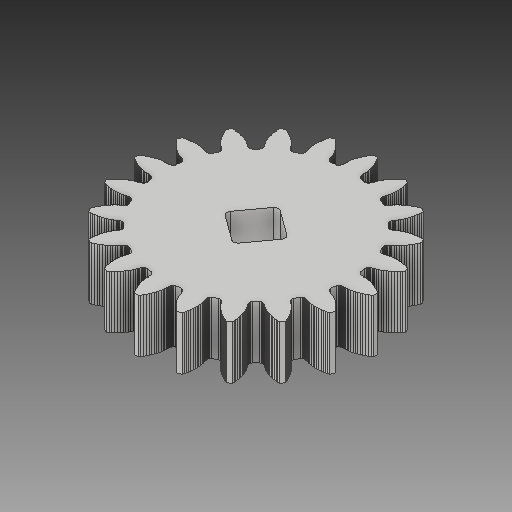
# Autodesk Inventor part: gear20
Saved by Autodesk Inventor 2019 (Build 230136000, 136)
## iProperties
Created: 2018-12-28
Part Number: gear20
Material: Generic
Document SubType Name: Modeling
Designer: Varga Daniel
Density: 1 g/cm^3
Appearance: Default
Sending System: SolidWorks 2018
Last Author: david
Last Saved: 2018-12-28
Author: Varga Daniel
Autodesk Inventor part; units mm, degrees
ref_plane "YZ Plane" through (0, 0, 0) normal (1, 0, 0) x (0, 1, 0)
ref_plane "XZ Plane" through (0, 0, 0) normal (0, 1, 0) x (-1, 0, 0)
ref_plane "XY Plane" through (0, 0, 0) normal (0, 0, 1) x (1, 0, 0)
sketch "Sketch1" plane through (0, 0, 0) normal (0, 1, 0) x (-1, 0, 0)
  line L0 (19.9269, 12.3554) -> (19.9815, 12.2461)
  line L1 (19.9815, 12.2461) -> (20.0271, 12.2067)
  line L2 (20.0271, 12.2067) -> (20.0711, 12.1796)
  line L3 (20.0711, 12.1796) -> (20.1144, 12.1591)
  line L4 (20.1144, 12.1591) -> (20.1571, 12.1432)
  line L5 (20.1571, 12.1432) -> (20.2414, 12.1206)
  line L6 (20.2414, 12.1206) -> (20.3248, 12.107)
  line L7 (20.3248, 12.107) -> (20.4075, 12.1)
  line L8 (20.4075, 12.1) -> (20.4897, 12.0984)
  line L9 (20.4897, 12.0984) -> (20.6534, 12.1025)
  line L10 (20.6534, 12.1025) -> (20.8187, 12.0882)
  line L11 (20.8187, 12.0882) -> (20.9851, 12.06)
  line L12 (20.9851, 12.06) -> (21.1522, 12.0208)
  line L13 (21.1522, 12.0208) -> (21.3198, 11.9721)
  line L14 (21.3198, 11.9721) -> (21.4876, 11.9147)
  line L15 (21.4876, 11.9147) -> (21.6554, 11.8491)
  line L16 (21.6554, 11.8491) -> (21.823, 11.7758)
  line L17 (21.823, 11.7758) -> (21.9904, 11.695)
  line L18 (21.9904, 11.695) -> (22.1573, 11.6069)
  line L19 (22.1573, 11.6069) -> (22.3236, 11.5119)
  line L20 (22.3236, 11.5119) -> (22.4478, 11.4361)
  line L21 (22.4478, 11.4361) -> (22.4478, 11.0137)
  line L22 (22.4478, 11.0137) -> (22.3236, 10.9379)
  line L23 (22.3236, 10.9379) -> (22.1573, 10.8429)
  line L24 (22.1573, 10.8429) -> (21.9904, 10.7549)
  line L25 (21.9904, 10.7549) -> (21.823, 10.6741)
  line L26 (21.823, 10.6741) -> (21.6554, 10.6007)
  line L27 (21.6554, 10.6007) -> (21.4876, 10.5351)
  line L28 (21.4876, 10.5351) -> (21.3198, 10.4777)
  line L29 (21.3198, 10.4777) -> (21.1522, 10.429)
  line L30 (21.1522, 10.429) -> (20.9851, 10.3898)
  line L31 (20.9851, 10.3898) -> (20.8187, 10.3616)
  line L32 (20.8187, 10.3616) -> (20.6534, 10.3473)
  line L33 (20.6534, 10.3473) -> (20.4897, 10.3514)
  line L34 (20.4897, 10.3514) -> (20.4075, 10.3498)
  line L35 (20.4075, 10.3498) -> (20.3248, 10.3428)
  line L36 (20.3248, 10.3428) -> (20.2414, 10.3292)
  line L37 (20.2414, 10.3292) -> (20.1571, 10.3066)
  line L38 (20.1571, 10.3066) -> (20.1144, 10.2907)
  line L39 (20.1144, 10.2907) -> (20.0711, 10.2703)
  line L40 (20.0711, 10.2703) -> (20.0271, 10.2431)
  line L41 (20.0271, 10.2431) -> (19.9815, 10.2037)
  line L42 (19.9815, 10.2037) -> (19.9269, 10.0944)
  line L43 (19.9269, 10.0944) -> (19.8503, 9.611)
  line L44 (19.8503, 9.611) -> (19.8685, 9.4902)
  line L45 (19.8685, 9.4902) -> (19.8997, 9.4386)
  line L46 (19.8997, 9.4386) -> (19.9332, 9.3992)
  line L47 (19.9332, 9.3992) -> (19.968, 9.3664)
  line L48 (19.968, 9.3664) -> (20.0037, 9.338)
  line L49 (20.0037, 9.338) -> (20.0769, 9.2905)
  line L50 (20.0769, 9.2905) -> (20.152, 9.2518)
  line L51 (20.152, 9.2518) -> (20.2285, 9.2196)
  line L52 (20.2285, 9.2196) -> (20.3062, 9.1927)
  line L53 (20.3062, 9.1927) -> (20.4631, 9.146)
  line L54 (20.4631, 9.146) -> (20.6159, 9.0813)
  line L55 (20.6159, 9.0813) -> (20.7655, 9.003)
  line L56 (20.7655, 9.003) -> (20.9123, 8.9141)
  line L57 (20.9123, 8.9141) -> (21.0566, 8.8161)
  line L58 (21.0566, 8.8161) -> (21.1984, 8.7096)
  line L59 (21.1984, 8.7096) -> (21.3378, 8.5954)
  line L60 (21.3378, 8.5954) -> (21.4746, 8.4738)
  line L61 (21.4746, 8.4738) -> (21.6088, 8.3452)
  line L62 (21.6088, 8.3452) -> (21.7403, 8.2099)
  line L63 (21.7403, 8.2099) -> (21.8691, 8.0681)
  line L64 (21.8691, 8.0681) -> (21.9638, 7.9577)
  line L65 (21.9638, 7.9577) -> (21.8333, 7.556)
  line L66 (21.8333, 7.556) -> (21.6917, 7.5223)
  line L67 (21.6917, 7.5223) -> (21.5042, 7.4833)
  line L68 (21.5042, 7.4833) -> (21.3183, 7.4511)
  line L69 (21.3183, 7.4511) -> (21.1341, 7.426)
  line L70 (21.1341, 7.426) -> (20.952, 7.4081)
  line L71 (20.952, 7.4081) -> (20.7721, 7.3976)
  line L72 (20.7721, 7.3976) -> (20.5948, 7.3948)
  line L73 (20.5948, 7.3948) -> (20.4204, 7.4002)
  line L74 (20.4204, 7.4002) -> (20.2493, 7.4146)
  line L75 (20.2493, 7.4146) -> (20.0824, 7.4392)
  line L76 (20.0824, 7.4392) -> (19.9207, 7.4767)
  line L77 (19.9207, 7.4767) -> (19.7663, 7.5312)
  line L78 (19.7663, 7.5312) -> (19.6877, 7.555)
  line L79 (19.6877, 7.555) -> (19.6068, 7.5739)
  line L80 (19.6068, 7.5739) -> (19.5233, 7.5868)
  line L81 (19.5233, 7.5868) -> (19.4362, 7.5914)
  line L82 (19.4362, 7.5914) -> (19.3906, 7.5894)
  line L83 (19.3906, 7.5894) -> (19.3432, 7.5834)
  line L84 (19.3432, 7.5834) -> (19.2929, 7.5712)
  line L85 (19.2929, 7.5712) -> (19.2373, 7.5477)
  line L86 (19.2373, 7.5477) -> (19.1516, 7.4607)
  line L87 (19.1516, 7.4607) -> (18.9294, 7.0246)
  line L88 (18.9294, 7.0246) -> (18.9094, 6.9041)
  line L89 (18.9094, 6.9041) -> (18.9231, 6.8454)
  line L90 (18.9231, 6.8454) -> (18.9428, 6.7976)
  line L91 (18.9428, 6.7976) -> (18.9657, 6.7556)
  line L92 (18.9657, 6.7556) -> (18.9909, 6.7176)
  line L93 (18.9909, 6.7176) -> (19.0459, 6.6498)
  line L94 (19.0459, 6.6498) -> (19.1054, 6.5898)
  line L95 (19.1054, 6.5898) -> (19.1682, 6.5355)
  line L96 (19.1682, 6.5355) -> (19.2337, 6.4859)
  line L97 (19.2337, 6.4859) -> (19.3685, 6.393)
  line L98 (19.3685, 6.393) -> (19.4938, 6.2843)
  line L99 (19.4938, 6.2843) -> (19.6119, 6.1636)
  line L100 (19.6119, 6.1636) -> (19.7241, 6.0337)
  line L101 (19.7241, 6.0337) -> (19.831, 5.8958)
  line L102 (19.831, 5.8958) -> (19.933, 5.7507)
  line L103 (19.933, 5.7507) -> (20.0302, 5.599)
  line L104 (20.0302, 5.599) -> (20.1228, 5.4411)
  line L105 (20.1228, 5.4411) -> (20.2107, 5.2774)
  line L106 (20.2107, 5.2774) -> (20.294, 5.1081)
  line L107 (20.294, 5.1081) -> (20.3726, 4.9334)
  line L108 (20.3726, 4.9334) -> (20.4286, 4.7991)
  line L109 (20.4286, 4.7991) -> (20.1803, 4.4574)
  line L110 (20.1803, 4.4574) -> (20.0353, 4.4691)
  line L111 (20.0353, 4.4691) -> (19.8449, 4.4899)
  line L112 (19.8449, 4.4899) -> (19.6581, 4.5168)
  line L113 (19.6581, 4.5168) -> (19.4752, 4.5498)
  line L114 (19.4752, 4.5498) -> (19.2964, 4.589)
  line L115 (19.2964, 4.589) -> (19.1221, 4.6346)
  line L116 (19.1221, 4.6346) -> (18.9526, 4.6868)
  line L117 (18.9526, 4.6868) -> (18.7885, 4.7459)
  line L118 (18.7885, 4.7459) -> (18.6302, 4.8124)
  line L119 (18.6302, 4.8124) -> (18.479, 4.8874)
  line L120 (18.479, 4.8874) -> (18.3369, 4.973)
  line L121 (18.3369, 4.973) -> (18.2069, 5.0725)
  line L122 (18.2069, 5.0725) -> (18.1394, 5.1195)
  line L123 (18.1394, 5.1195) -> (18.0684, 5.1625)
  line L124 (18.0684, 5.1625) -> (17.9929, 5.2005)
  line L125 (17.9929, 5.2005) -> (17.9114, 5.2318)
  line L126 (17.9114, 5.2318) -> (17.8675, 5.244)
  line L127 (17.8675, 5.244) -> (17.8205, 5.2529)
  line L128 (17.8205, 5.2529) -> (17.7689, 5.2568)
  line L129 (17.7689, 5.2568) -> (17.7089, 5.2517)
  line L130 (17.7089, 5.2517) -> (17.6005, 5.1954)
  line L131 (17.6005, 5.1954) -> (17.2544, 4.8494)
  line L132 (17.2544, 4.8494) -> (17.1981, 4.7409)
  line L133 (17.1981, 4.7409) -> (17.193, 4.6809)
  line L134 (17.193, 4.6809) -> (17.1969, 4.6293)
  line L135 (17.1969, 4.6293) -> (17.2058, 4.5823)
  line L136 (17.2058, 4.5823) -> (17.218, 4.5384)
  line L137 (17.218, 4.5384) -> (17.2493, 4.4569)
  line L138 (17.2493, 4.4569) -> (17.2873, 4.3814)
  line L139 (17.2873, 4.3814) -> (17.3303, 4.3104)
  line L140 (17.3303, 4.3104) -> (17.3773, 4.2429)
  line L141 (17.3773, 4.2429) -> (17.4768, 4.113)
  line L142 (17.4768, 4.113) -> (17.5624, 3.9708)
  line L143 (17.5624, 3.9708) -> (17.6374, 3.8196)
  line L144 (17.6374, 3.8196) -> (17.7039, 3.6614)
  line L145 (17.7039, 3.6614) -> (17.763, 3.4972)
  line L146 (17.763, 3.4972) -> (17.8152, 3.3277)
  line L147 (17.8152, 3.3277) -> (17.8608, 3.1534)
  line L148 (17.8608, 3.1534) -> (17.9, 2.9746)
  line L149 (17.9, 2.9746) -> (17.933, 2.7917)
  line L150 (17.933, 2.7917) -> (17.9599, 2.6049)
  line L151 (17.9599, 2.6049) -> (17.9807, 2.4145)
  line L152 (17.9807, 2.4145) -> (17.9924, 2.2695)
  line L153 (17.9924, 2.2695) -> (17.6507, 2.0213)
  line L154 (17.6507, 2.0213) -> (17.5164, 2.0772)
  line L155 (17.5164, 2.0772) -> (17.3418, 2.1559)
  line L156 (17.3418, 2.1559) -> (17.1725, 2.2391)
  line L157 (17.1725, 2.2391) -> (17.0087, 2.327)
  line L158 (17.0087, 2.327) -> (16.8508, 2.4196)
  line L159 (16.8508, 2.4196) -> (16.6991, 2.5168)
  line L160 (16.6991, 2.5168) -> (16.554, 2.6188)
  line L161 (16.554, 2.6188) -> (16.4161, 2.7257)
  line L162 (16.4161, 2.7257) -> (16.2862, 2.8379)
  line L163 (16.2862, 2.8379) -> (16.1656, 2.956)
  line L164 (16.1656, 2.956) -> (16.0568, 3.0813)
  line L165 (16.0568, 3.0813) -> (15.964, 3.2161)
  line L166 (15.964, 3.2161) -> (15.9143, 3.2816)
  line L167 (15.9143, 3.2816) -> (15.8601, 3.3444)
  line L168 (15.8601, 3.3444) -> (15.8, 3.4039)
  line L169 (15.8, 3.4039) -> (15.7322, 3.4589)
  line L170 (15.7322, 3.4589) -> (15.6942, 3.4841)
  line L171 (15.6942, 3.4841) -> (15.6523, 3.507)
  line L172 (15.6523, 3.507) -> (15.6044, 3.5267)
  line L173 (15.6044, 3.5267) -> (15.5457, 3.5404)
  line L174 (15.5457, 3.5404) -> (15.4252, 3.5204)
  line L175 (15.4252, 3.5204) -> (14.9891, 3.2982)
  line L176 (14.9891, 3.2982) -> (14.9021, 3.2125)
  line L177 (14.9021, 3.2125) -> (14.8787, 3.1569)
  line L178 (14.8787, 3.1569) -> (14.8665, 3.1067)
  line L179 (14.8665, 3.1067) -> (14.8604, 3.0592)
  line L180 (14.8604, 3.0592) -> (14.8584, 3.0137)
  line L181 (14.8584, 3.0137) -> (14.863, 2.9265)
  line L182 (14.863, 2.9265) -> (14.8759, 2.843)
  line L183 (14.8759, 2.843) -> (14.8948, 2.7622)
  line L184 (14.8948, 2.7622) -> (14.9186, 2.6835)
  line L185 (14.9186, 2.6835) -> (14.9731, 2.5291)
  line L186 (14.9731, 2.5291) -> (15.0106, 2.3675)
  line L187 (15.0106, 2.3675) -> (15.0352, 2.2005)
  line L188 (15.0352, 2.2005) -> (15.0496, 2.0294)
  line L189 (15.0496, 2.0294) -> (15.055, 1.855)
  line L190 (15.055, 1.855) -> (15.0523, 1.6777)
  line L191 (15.0523, 1.6777) -> (15.0418, 1.4978)
  line L192 (15.0418, 1.4978) -> (15.0238, 1.3157)
  line L193 (15.0238, 1.3157) -> (14.9987, 1.1315)
  line L194 (14.9987, 1.1315) -> (14.9665, 0.9456)
  line L195 (14.9665, 0.9456) -> (14.9275, 0.7581)
  line L196 (14.9275, 0.7581) -> (14.8938, 0.6165)
  line L197 (14.8938, 0.6165) -> (14.4922, 0.486)
  line L198 (14.4922, 0.486) -> (14.3817, 0.5807)
  line L199 (14.3817, 0.5807) -> (14.2399, 0.7095)
  line L200 (14.2399, 0.7095) -> (14.1046, 0.841)
  line L201 (14.1046, 0.841) -> (13.976, 0.9752)
  line L202 (13.976, 0.9752) -> (13.8544, 1.112)
  line L203 (13.8544, 1.112) -> (13.7402, 1.2514)
  line L204 (13.7402, 1.2514) -> (13.6338, 1.3932)
  line L205 (13.6338, 1.3932) -> (13.5357, 1.5375)
  line L206 (13.5357, 1.5375) -> (13.4468, 1.6844)
  line L207 (13.4468, 1.6844) -> (13.3685, 1.8339)
  line L208 (13.3685, 1.8339) -> (13.3038, 1.9867)
  line L209 (13.3038, 1.9867) -> (13.2572, 2.1436)
  line L210 (13.2572, 2.1436) -> (13.2302, 2.2213)
  line L211 (13.2302, 2.2213) -> (13.198, 2.2978)
  line L212 (13.198, 2.2978) -> (13.1593, 2.3729)
  line L213 (13.1593, 2.3729) -> (13.1118, 2.4461)
  line L214 (13.1118, 2.4461) -> (13.0834, 2.4818)
  line L215 (13.0834, 2.4818) -> (13.0506, 2.5166)
  line L216 (13.0506, 2.5166) -> (13.0112, 2.5502)
  line L217 (13.0112, 2.5502) -> (12.9596, 2.5813)
  line L218 (12.9596, 2.5813) -> (12.8388, 2.5995)
  line L219 (12.8388, 2.5995) -> (12.3554, 2.5229)
  line L220 (12.3554, 2.5229) -> (12.2461, 2.4683)
  line L221 (12.2461, 2.4683) -> (12.2067, 2.4227)
  line L222 (12.2067, 2.4227) -> (12.1796, 2.3787)
  line L223 (12.1796, 2.3787) -> (12.1591, 2.3354)
  line L224 (12.1591, 2.3354) -> (12.1432, 2.2927)
  line L225 (12.1432, 2.2927) -> (12.1206, 2.2084)
  line L226 (12.1206, 2.2084) -> (12.107, 2.125)
  line L227 (12.107, 2.125) -> (12.1, 2.0423)
  line L228 (12.1, 2.0423) -> (12.0984, 1.9601)
  line L229 (12.0984, 1.9601) -> (12.1025, 1.7965)
  line L230 (12.1025, 1.7965) -> (12.0882, 1.6311)
  line L231 (12.0882, 1.6311) -> (12.06, 1.4647)
  line L232 (12.06, 1.4647) -> (12.0208, 1.2976)
  line L233 (12.0208, 1.2976) -> (11.9721, 1.13)
  line L234 (11.9721, 1.13) -> (11.9147, 0.9623)
  line L235 (11.9147, 0.9623) -> (11.8491, 0.7944)
  line L236 (11.8491, 0.7944) -> (11.7758, 0.6268)
  line L237 (11.7758, 0.6268) -> (11.695, 0.4594)
  line L238 (11.695, 0.4594) -> (11.6069, 0.2925)
  line L239 (11.6069, 0.2925) -> (11.5119, 0.1262)
  line L240 (11.5119, 0.1262) -> (11.4361, 0.002)
  line L241 (11.4361, 0.002) -> (11.0137, 0.002)
  line L242 (11.0137, 0.002) -> (10.9379, 0.1262)
  line L243 (10.9379, 0.1262) -> (10.8429, 0.2925)
  line L244 (10.8429, 0.2925) -> (10.7549, 0.4594)
  line L245 (10.7549, 0.4594) -> (10.6741, 0.6268)
  line L246 (10.6741, 0.6268) -> (10.6007, 0.7944)
  line L247 (10.6007, 0.7944) -> (10.5351, 0.9623)
  line L248 (10.5351, 0.9623) -> (10.4777, 1.13)
  line L249 (10.4777, 1.13) -> (10.429, 1.2976)
  line L250 (10.429, 1.2976) -> (10.3898, 1.4647)
  line L251 (10.3898, 1.4647) -> (10.3616, 1.6311)
  line L252 (10.3616, 1.6311) -> (10.3473, 1.7965)
  line L253 (10.3473, 1.7965) -> (10.3514, 1.9601)
  line L254 (10.3514, 1.9601) -> (10.3498, 2.0423)
  line L255 (10.3498, 2.0423) -> (10.3428, 2.125)
  line L256 (10.3428, 2.125) -> (10.3292, 2.2084)
  line L257 (10.3292, 2.2084) -> (10.3066, 2.2927)
  line L258 (10.3066, 2.2927) -> (10.2907, 2.3354)
  line L259 (10.2907, 2.3354) -> (10.2703, 2.3787)
  line L260 (10.2703, 2.3787) -> (10.2431, 2.4227)
  line L261 (10.2431, 2.4227) -> (10.2037, 2.4683)
  line L262 (10.2037, 2.4683) -> (10.0944, 2.5229)
  line L263 (10.0944, 2.5229) -> (9.611, 2.5995)
  line L264 (9.611, 2.5995) -> (9.4902, 2.5813)
  line L265 (9.4902, 2.5813) -> (9.4386, 2.5502)
  line L266 (9.4386, 2.5502) -> (9.3992, 2.5166)
  line L267 (9.3992, 2.5166) -> (9.3664, 2.4818)
  line L268 (9.3664, 2.4818) -> (9.338, 2.4461)
  line L269 (9.338, 2.4461) -> (9.2905, 2.3729)
  line L270 (9.2905, 2.3729) -> (9.2518, 2.2978)
  line L271 (9.2518, 2.2978) -> (9.2196, 2.2213)
  line L272 (9.2196, 2.2213) -> (9.1927, 2.1436)
  line L273 (9.1927, 2.1436) -> (9.146, 1.9867)
  line L274 (9.146, 1.9867) -> (9.0813, 1.8339)
  line L275 (9.0813, 1.8339) -> (9.003, 1.6844)
  line L276 (9.003, 1.6844) -> (8.9141, 1.5375)
  line L277 (8.9141, 1.5375) -> (8.8161, 1.3932)
  line L278 (8.8161, 1.3932) -> (8.7096, 1.2514)
  line L279 (8.7096, 1.2514) -> (8.5954, 1.112)
  line L280 (8.5954, 1.112) -> (8.4738, 0.9752)
  line L281 (8.4738, 0.9752) -> (8.3452, 0.841)
  line L282 (8.3452, 0.841) -> (8.2099, 0.7095)
  line L283 (8.2099, 0.7095) -> (8.0681, 0.5807)
  line L284 (8.0681, 0.5807) -> (7.9577, 0.486)
  line L285 (7.9577, 0.486) -> (7.556, 0.6165)
  line L286 (7.556, 0.6165) -> (7.5223, 0.7581)
  line L287 (7.5223, 0.7581) -> (7.4833, 0.9456)
  line L288 (7.4833, 0.9456) -> (7.4511, 1.1315)
  line L289 (7.4511, 1.1315) -> (7.426, 1.3157)
  line L290 (7.426, 1.3157) -> (7.4081, 1.4978)
  line L291 (7.4081, 1.4978) -> (7.3976, 1.6777)
  line L292 (7.3976, 1.6777) -> (7.3948, 1.855)
  line L293 (7.3948, 1.855) -> (7.4002, 2.0294)
  line L294 (7.4002, 2.0294) -> (7.4146, 2.2005)
  line L295 (7.4146, 2.2005) -> (7.4392, 2.3675)
  line L296 (7.4392, 2.3675) -> (7.4767, 2.5291)
  line L297 (7.4767, 2.5291) -> (7.5312, 2.6835)
  line L298 (7.5312, 2.6835) -> (7.555, 2.7622)
  line L299 (7.555, 2.7622) -> (7.5739, 2.843)
  line L300 (7.5739, 2.843) -> (7.5868, 2.9265)
  line L301 (7.5868, 2.9265) -> (7.5914, 3.0137)
  line L302 (7.5914, 3.0137) -> (7.5894, 3.0592)
  line L303 (7.5894, 3.0592) -> (7.5834, 3.1067)
  line L304 (7.5834, 3.1067) -> (7.5712, 3.1569)
  line L305 (7.5712, 3.1569) -> (7.5477, 3.2125)
  line L306 (7.5477, 3.2125) -> (7.4607, 3.2982)
  line L307 (7.4607, 3.2982) -> (7.0246, 3.5204)
  line L308 (7.0246, 3.5204) -> (6.9041, 3.5404)
  line L309 (6.9041, 3.5404) -> (6.8454, 3.5267)
  line L310 (6.8454, 3.5267) -> (6.7976, 3.507)
  line L311 (6.7976, 3.507) -> (6.7556, 3.4841)
  line L312 (6.7556, 3.4841) -> (6.7176, 3.4589)
  line L313 (6.7176, 3.4589) -> (6.6498, 3.4039)
  line L314 (6.6498, 3.4039) -> (6.5898, 3.3444)
  line L315 (6.5898, 3.3444) -> (6.5355, 3.2816)
  line L316 (6.5355, 3.2816) -> (6.4859, 3.2161)
  line L317 (6.4859, 3.2161) -> (6.393, 3.0813)
  line L318 (6.393, 3.0813) -> (6.2843, 2.956)
  line L319 (6.2843, 2.956) -> (6.1636, 2.8379)
  line L320 (6.1636, 2.8379) -> (6.0337, 2.7257)
  line L321 (6.0337, 2.7257) -> (5.8958, 2.6188)
  line L322 (5.8958, 2.6188) -> (5.7507, 2.5168)
  line L323 (5.7507, 2.5168) -> (5.599, 2.4196)
  line L324 (5.599, 2.4196) -> (5.4411, 2.327)
  line L325 (5.4411, 2.327) -> (5.2774, 2.2391)
  line L326 (5.2774, 2.2391) -> (5.1081, 2.1559)
  line L327 (5.1081, 2.1559) -> (4.9334, 2.0772)
  line L328 (4.9334, 2.0772) -> (4.7991, 2.0213)
  line L329 (4.7991, 2.0213) -> (4.4574, 2.2695)
  line L330 (4.4574, 2.2695) -> (4.4691, 2.4145)
  line L331 (4.4691, 2.4145) -> (4.4899, 2.6049)
  line L332 (4.4899, 2.6049) -> (4.5168, 2.7917)
  line L333 (4.5168, 2.7917) -> (4.5498, 2.9746)
  line L334 (4.5498, 2.9746) -> (4.589, 3.1534)
  line L335 (4.589, 3.1534) -> (4.6346, 3.3277)
  line L336 (4.6346, 3.3277) -> (4.6868, 3.4972)
  line L337 (4.6868, 3.4972) -> (4.7459, 3.6614)
  line L338 (4.7459, 3.6614) -> (4.8124, 3.8196)
  line L339 (4.8124, 3.8196) -> (4.8874, 3.9708)
  line L340 (4.8874, 3.9708) -> (4.973, 4.113)
  line L341 (4.973, 4.113) -> (5.0725, 4.2429)
  line L342 (5.0725, 4.2429) -> (5.1195, 4.3104)
  line L343 (5.1195, 4.3104) -> (5.1625, 4.3814)
  line L344 (5.1625, 4.3814) -> (5.2005, 4.4569)
  line L345 (5.2005, 4.4569) -> (5.2318, 4.5384)
  line L346 (5.2318, 4.5384) -> (5.244, 4.5823)
  line L347 (5.244, 4.5823) -> (5.2529, 4.6293)
  line L348 (5.2529, 4.6293) -> (5.2568, 4.6809)
  line L349 (5.2568, 4.6809) -> (5.2517, 4.7409)
  line L350 (5.2517, 4.7409) -> (5.1954, 4.8494)
  line L351 (5.1954, 4.8494) -> (4.8494, 5.1954)
  line L352 (4.8494, 5.1954) -> (4.7409, 5.2517)
  line L353 (4.7409, 5.2517) -> (4.6809, 5.2568)
  line L354 (4.6809, 5.2568) -> (4.6293, 5.2529)
  line L355 (4.6293, 5.2529) -> (4.5823, 5.244)
  line L356 (4.5823, 5.244) -> (4.5384, 5.2318)
  line L357 (4.5384, 5.2318) -> (4.4569, 5.2005)
  line L358 (4.4569, 5.2005) -> (4.3814, 5.1625)
  line L359 (4.3814, 5.1625) -> (4.3104, 5.1195)
  line L360 (4.3104, 5.1195) -> (4.2429, 5.0725)
  line L361 (4.2429, 5.0725) -> (4.113, 4.973)
  line L362 (4.113, 4.973) -> (3.9708, 4.8874)
  line L363 (3.9708, 4.8874) -> (3.8196, 4.8124)
  line L364 (3.8196, 4.8124) -> (3.6614, 4.7459)
  line L365 (3.6614, 4.7459) -> (3.4972, 4.6868)
  line L366 (3.4972, 4.6868) -> (3.3277, 4.6346)
  line L367 (3.3277, 4.6346) -> (3.1534, 4.589)
  line L368 (3.1534, 4.589) -> (2.9746, 4.5498)
  line L369 (2.9746, 4.5498) -> (2.7917, 4.5168)
  line L370 (2.7917, 4.5168) -> (2.6049, 4.4899)
  line L371 (2.6049, 4.4899) -> (2.4145, 4.4691)
  line L372 (2.4145, 4.4691) -> (2.2695, 4.4574)
  line L373 (2.2695, 4.4574) -> (2.0213, 4.7991)
  line L374 (2.0213, 4.7991) -> (2.0772, 4.9334)
  line L375 (2.0772, 4.9334) -> (2.1559, 5.1081)
  line L376 (2.1559, 5.1081) -> (2.2391, 5.2774)
  line L377 (2.2391, 5.2774) -> (2.327, 5.4411)
  line L378 (2.327, 5.4411) -> (2.4196, 5.599)
  line L379 (2.4196, 5.599) -> (2.5168, 5.7507)
  line L380 (2.5168, 5.7507) -> (2.6188, 5.8958)
  line L381 (2.6188, 5.8958) -> (2.7257, 6.0337)
  line L382 (2.7257, 6.0337) -> (2.8379, 6.1636)
  line L383 (2.8379, 6.1636) -> (2.956, 6.2843)
  line L384 (2.956, 6.2843) -> (3.0813, 6.393)
  line L385 (3.0813, 6.393) -> (3.2161, 6.4859)
  line L386 (3.2161, 6.4859) -> (3.2816, 6.5355)
  line L387 (3.2816, 6.5355) -> (3.3444, 6.5898)
  line L388 (3.3444, 6.5898) -> (3.4039, 6.6498)
  line L389 (3.4039, 6.6498) -> (3.4589, 6.7176)
  line L390 (3.4589, 6.7176) -> (3.4841, 6.7556)
  line L391 (3.4841, 6.7556) -> (3.507, 6.7976)
  line L392 (3.507, 6.7976) -> (3.5267, 6.8454)
  line L393 (3.5267, 6.8454) -> (3.5404, 6.9041)
  line L394 (3.5404, 6.9041) -> (3.5204, 7.0246)
  line L395 (3.5204, 7.0246) -> (3.2982, 7.4607)
  line L396 (3.2982, 7.4607) -> (3.2125, 7.5477)
  line L397 (3.2125, 7.5477) -> (3.1569, 7.5712)
  line L398 (3.1569, 7.5712) -> (3.1067, 7.5834)
  line L399 (3.1067, 7.5834) -> (3.0592, 7.5894)
  line L400 (3.0592, 7.5894) -> (3.0137, 7.5914)
  line L401 (3.0137, 7.5914) -> (2.9265, 7.5868)
  line L402 (2.9265, 7.5868) -> (2.843, 7.5739)
  line L403 (2.843, 7.5739) -> (2.7622, 7.555)
  line L404 (2.7622, 7.555) -> (2.6835, 7.5312)
  line L405 (2.6835, 7.5312) -> (2.5291, 7.4767)
  line L406 (2.5291, 7.4767) -> (2.3675, 7.4392)
  line L407 (2.3675, 7.4392) -> (2.2005, 7.4146)
  line L408 (2.2005, 7.4146) -> (2.0294, 7.4002)
  line L409 (2.0294, 7.4002) -> (1.855, 7.3948)
  line L410 (1.855, 7.3948) -> (1.6777, 7.3976)
  line L411 (1.6777, 7.3976) -> (1.4978, 7.4081)
  line L412 (1.4978, 7.4081) -> (1.3157, 7.426)
  line L413 (1.3157, 7.426) -> (1.1315, 7.4511)
  line L414 (1.1315, 7.4511) -> (0.9456, 7.4833)
  line L415 (0.9456, 7.4833) -> (0.7581, 7.5223)
  line L416 (0.7581, 7.5223) -> (0.6165, 7.556)
  line L417 (0.6165, 7.556) -> (0.486, 7.9577)
  line L418 (0.486, 7.9577) -> (0.5807, 8.0681)
  line L419 (0.5807, 8.0681) -> (0.7095, 8.2099)
  line L420 (0.7095, 8.2099) -> (0.841, 8.3452)
  line L421 (0.841, 8.3452) -> (0.9752, 8.4738)
  line L422 (0.9752, 8.4738) -> (1.112, 8.5954)
  line L423 (1.112, 8.5954) -> (1.2514, 8.7096)
  line L424 (1.2514, 8.7096) -> (1.3932, 8.8161)
  line L425 (1.3932, 8.8161) -> (1.5375, 8.9141)
  line L426 (1.5375, 8.9141) -> (1.6844, 9.003)
  line L427 (1.6844, 9.003) -> (1.8339, 9.0813)
  line L428 (1.8339, 9.0813) -> (1.9867, 9.146)
  line L429 (1.9867, 9.146) -> (2.1436, 9.1927)
  line L430 (2.1436, 9.1927) -> (2.2213, 9.2196)
  line L431 (2.2213, 9.2196) -> (2.2978, 9.2518)
  line L432 (2.2978, 9.2518) -> (2.3729, 9.2905)
  line L433 (2.3729, 9.2905) -> (2.4461, 9.338)
  line L434 (2.4461, 9.338) -> (2.4818, 9.3664)
  line L435 (2.4818, 9.3664) -> (2.5166, 9.3992)
  line L436 (2.5166, 9.3992) -> (2.5502, 9.4386)
  line L437 (2.5502, 9.4386) -> (2.5813, 9.4902)
  line L438 (2.5813, 9.4902) -> (2.5995, 9.611)
  line L439 (2.5995, 9.611) -> (2.5229, 10.0944)
  line L440 (2.5229, 10.0944) -> (2.4683, 10.2037)
  line L441 (2.4683, 10.2037) -> (2.4227, 10.2431)
  line L442 (2.4227, 10.2431) -> (2.3787, 10.2703)
  line L443 (2.3787, 10.2703) -> (2.3354, 10.2907)
  line L444 (2.3354, 10.2907) -> (2.2927, 10.3066)
  line L445 (2.2927, 10.3066) -> (2.2084, 10.3292)
  line L446 (2.2084, 10.3292) -> (2.125, 10.3428)
  line L447 (2.125, 10.3428) -> (2.0423, 10.3498)
  line L448 (2.0423, 10.3498) -> (1.9601, 10.3514)
  line L449 (1.9601, 10.3514) -> (1.7965, 10.3473)
  line L450 (1.7965, 10.3473) -> (1.6311, 10.3616)
  line L451 (1.6311, 10.3616) -> (1.4647, 10.3898)
  line L452 (1.4647, 10.3898) -> (1.2976, 10.429)
  line L453 (1.2976, 10.429) -> (1.13, 10.4777)
  line L454 (1.13, 10.4777) -> (0.9623, 10.5351)
  line L455 (0.9623, 10.5351) -> (0.7944, 10.6007)
  line L456 (0.7944, 10.6007) -> (0.6268, 10.6741)
  line L457 (0.6268, 10.6741) -> (0.4594, 10.7549)
  line L458 (0.4594, 10.7549) -> (0.2925, 10.8429)
  line L459 (0.2925, 10.8429) -> (0.1262, 10.9379)
  line L460 (0.1262, 10.9379) -> (0.002, 11.0137)
  line L461 (0.002, 11.0137) -> (0.002, 11.4361)
  line L462 (0.002, 11.4361) -> (0.1262, 11.5119)
  line L463 (0.1262, 11.5119) -> (0.2925, 11.6069)
  line L464 (0.2925, 11.6069) -> (0.4594, 11.695)
  line L465 (0.4594, 11.695) -> (0.6268, 11.7758)
  line L466 (0.6268, 11.7758) -> (0.7944, 11.8491)
  line L467 (0.7944, 11.8491) -> (0.9623, 11.9147)
  line L468 (0.9623, 11.9147) -> (1.13, 11.9721)
  line L469 (1.13, 11.9721) -> (1.2976, 12.0208)
  line L470 (1.2976, 12.0208) -> (1.4647, 12.06)
  line L471 (1.4647, 12.06) -> (1.6311, 12.0882)
  line L472 (1.6311, 12.0882) -> (1.7965, 12.1025)
  line L473 (1.7965, 12.1025) -> (1.9601, 12.0984)
  line L474 (1.9601, 12.0984) -> (2.0423, 12.1)
  line L475 (2.0423, 12.1) -> (2.125, 12.107)
  line L476 (2.125, 12.107) -> (2.2084, 12.1206)
  line L477 (2.2084, 12.1206) -> (2.2927, 12.1432)
  line L478 (2.2927, 12.1432) -> (2.3354, 12.1591)
  line L479 (2.3354, 12.1591) -> (2.3787, 12.1796)
  line L480 (2.3787, 12.1796) -> (2.4227, 12.2067)
  line L481 (2.4227, 12.2067) -> (2.4683, 12.2461)
  line L482 (2.4683, 12.2461) -> (2.5229, 12.3554)
  line L483 (2.5229, 12.3554) -> (2.5995, 12.8388)
  line L484 (2.5995, 12.8388) -> (2.5813, 12.9596)
  line L485 (2.5813, 12.9596) -> (2.5502, 13.0112)
  line L486 (2.5502, 13.0112) -> (2.5166, 13.0506)
  line L487 (2.5166, 13.0506) -> (2.4818, 13.0834)
  line L488 (2.4818, 13.0834) -> (2.4461, 13.1118)
  line L489 (2.4461, 13.1118) -> (2.3729, 13.1593)
  line L490 (2.3729, 13.1593) -> (2.2978, 13.198)
  line L491 (2.2978, 13.198) -> (2.2213, 13.2302)
  line L492 (2.2213, 13.2302) -> (2.1436, 13.2572)
  line L493 (2.1436, 13.2572) -> (1.9867, 13.3038)
  line L494 (1.9867, 13.3038) -> (1.8339, 13.3685)
  line L495 (1.8339, 13.3685) -> (1.6844, 13.4468)
  line L496 (1.6844, 13.4468) -> (1.5375, 13.5357)
  line L497 (1.5375, 13.5357) -> (1.3932, 13.6338)
  line L498 (1.3932, 13.6338) -> (1.2514, 13.7402)
  line L499 (1.2514, 13.7402) -> (1.112, 13.8544)
  line L500 (1.112, 13.8544) -> (0.9752, 13.976)
  line L501 (0.9752, 13.976) -> (0.841, 14.1046)
  line L502 (0.841, 14.1046) -> (0.7095, 14.2399)
  line L503 (0.7095, 14.2399) -> (0.5807, 14.3817)
  line L504 (0.5807, 14.3817) -> (0.486, 14.4922)
  line L505 (0.486, 14.4922) -> (0.6165, 14.8938)
  line L506 (0.6165, 14.8938) -> (0.7581, 14.9275)
  line L507 (0.7581, 14.9275) -> (0.9456, 14.9665)
  line L508 (0.9456, 14.9665) -> (1.1315, 14.9987)
  line L509 (1.1315, 14.9987) -> (1.3157, 15.0238)
  line L510 (1.3157, 15.0238) -> (1.4978, 15.0418)
  line L511 (1.4978, 15.0418) -> (1.6777, 15.0523)
  line L512 (1.6777, 15.0523) -> (1.855, 15.055)
  line L513 (1.855, 15.055) -> (2.0294, 15.0496)
  line L514 (2.0294, 15.0496) -> (2.2005, 15.0352)
  line L515 (2.2005, 15.0352) -> (2.3675, 15.0106)
  line L516 (2.3675, 15.0106) -> (2.5291, 14.9731)
  line L517 (2.5291, 14.9731) -> (2.6835, 14.9186)
  line L518 (2.6835, 14.9186) -> (2.7622, 14.8948)
  line L519 (2.7622, 14.8948) -> (2.843, 14.8759)
  line L520 (2.843, 14.8759) -> (2.9265, 14.863)
  line L521 (2.9265, 14.863) -> (3.0137, 14.8584)
  line L522 (3.0137, 14.8584) -> (3.0592, 14.8604)
  line L523 (3.0592, 14.8604) -> (3.1067, 14.8665)
  line L524 (3.1067, 14.8665) -> (3.1569, 14.8787)
  line L525 (3.1569, 14.8787) -> (3.2125, 14.9021)
  line L526 (3.2125, 14.9021) -> (3.2982, 14.9891)
  line L527 (3.2982, 14.9891) -> (3.5204, 15.4252)
  line L528 (3.5204, 15.4252) -> (3.5404, 15.5457)
  line L529 (3.5404, 15.5457) -> (3.5267, 15.6044)
  line L530 (3.5267, 15.6044) -> (3.507, 15.6523)
  line L531 (3.507, 15.6523) -> (3.4841, 15.6942)
  line L532 (3.4841, 15.6942) -> (3.4589, 15.7322)
  line L533 (3.4589, 15.7322) -> (3.4039, 15.8)
  line L534 (3.4039, 15.8) -> (3.3444, 15.8601)
  line L535 (3.3444, 15.8601) -> (3.2816, 15.9143)
  line L536 (3.2816, 15.9143) -> (3.2161, 15.964)
  line L537 (3.2161, 15.964) -> (3.0813, 16.0568)
  line L538 (3.0813, 16.0568) -> (2.956, 16.1656)
  line L539 (2.956, 16.1656) -> (2.8379, 16.2862)
  line L540 (2.8379, 16.2862) -> (2.7257, 16.4161)
  line L541 (2.7257, 16.4161) -> (2.6188, 16.554)
  line L542 (2.6188, 16.554) -> (2.5168, 16.6991)
  line L543 (2.5168, 16.6991) -> (2.4196, 16.8508)
  line L544 (2.4196, 16.8508) -> (2.327, 17.0087)
  line L545 (2.327, 17.0087) -> (2.2391, 17.1725)
  line L546 (2.2391, 17.1725) -> (2.1559, 17.3418)
  line L547 (2.1559, 17.3418) -> (2.0772, 17.5164)
  line L548 (2.0772, 17.5164) -> (2.0213, 17.6507)
  line L549 (2.0213, 17.6507) -> (2.2695, 17.9924)
  line L550 (2.2695, 17.9924) -> (2.4145, 17.9807)
  line L551 (2.4145, 17.9807) -> (2.6049, 17.9599)
  line L552 (2.6049, 17.9599) -> (2.7917, 17.933)
  line L553 (2.7917, 17.933) -> (2.9746, 17.9)
  line L554 (2.9746, 17.9) -> (3.1534, 17.8608)
  line L555 (3.1534, 17.8608) -> (3.3277, 17.8152)
  line L556 (3.3277, 17.8152) -> (3.4972, 17.763)
  line L557 (3.4972, 17.763) -> (3.6614, 17.7039)
  line L558 (3.6614, 17.7039) -> (3.8196, 17.6374)
  line L559 (3.8196, 17.6374) -> (3.9708, 17.5624)
  line L560 (3.9708, 17.5624) -> (4.113, 17.4768)
  line L561 (4.113, 17.4768) -> (4.2429, 17.3773)
  line L562 (4.2429, 17.3773) -> (4.3104, 17.3303)
  line L563 (4.3104, 17.3303) -> (4.3814, 17.2873)
  line L564 (4.3814, 17.2873) -> (4.4569, 17.2493)
  line L565 (4.4569, 17.2493) -> (4.5384, 17.218)
  line L566 (4.5384, 17.218) -> (4.5823, 17.2058)
  line L567 (4.5823, 17.2058) -> (4.6293, 17.1969)
  line L568 (4.6293, 17.1969) -> (4.6809, 17.193)
  line L569 (4.6809, 17.193) -> (4.7409, 17.1981)
  line L570 (4.7409, 17.1981) -> (4.8494, 17.2544)
  line L571 (4.8494, 17.2544) -> (5.1954, 17.6005)
  line L572 (5.1954, 17.6005) -> (5.2517, 17.7089)
  line L573 (5.2517, 17.7089) -> (5.2568, 17.7689)
  line L574 (5.2568, 17.7689) -> (5.2529, 17.8205)
  line L575 (5.2529, 17.8205) -> (5.244, 17.8675)
  line L576 (5.244, 17.8675) -> (5.2318, 17.9114)
  line L577 (5.2318, 17.9114) -> (5.2005, 17.9929)
  line L578 (5.2005, 17.9929) -> (5.1625, 18.0684)
  line L579 (5.1625, 18.0684) -> (5.1195, 18.1394)
  line L580 (5.1195, 18.1394) -> (5.0725, 18.2069)
  line L581 (5.0725, 18.2069) -> (4.973, 18.3369)
  line L582 (4.973, 18.3369) -> (4.8874, 18.479)
  line L583 (4.8874, 18.479) -> (4.8124, 18.6302)
  line L584 (4.8124, 18.6302) -> (4.7459, 18.7885)
  line L585 (4.7459, 18.7885) -> (4.6868, 18.9526)
  line L586 (4.6868, 18.9526) -> (4.6346, 19.1221)
  line L587 (4.6346, 19.1221) -> (4.589, 19.2964)
  line L588 (4.589, 19.2964) -> (4.5498, 19.4752)
  line L589 (4.5498, 19.4752) -> (4.5168, 19.6581)
  line L590 (4.5168, 19.6581) -> (4.4899, 19.8449)
  line L591 (4.4899, 19.8449) -> (4.4691, 20.0353)
  line L592 (4.4691, 20.0353) -> (4.4574, 20.1803)
  line L593 (4.4574, 20.1803) -> (4.7991, 20.4286)
  line L594 (4.7991, 20.4286) -> (4.9334, 20.3726)
  line L595 (4.9334, 20.3726) -> (5.1081, 20.294)
  line L596 (5.1081, 20.294) -> (5.2774, 20.2107)
  line L597 (5.2774, 20.2107) -> (5.4411, 20.1228)
  line L598 (5.4411, 20.1228) -> (5.599, 20.0302)
  line L599 (5.599, 20.0302) -> (5.7507, 19.933)
  line L600 (5.7507, 19.933) -> (5.8958, 19.831)
  line L601 (5.8958, 19.831) -> (6.0337, 19.7241)
  line L602 (6.0337, 19.7241) -> (6.1636, 19.6119)
  line L603 (6.1636, 19.6119) -> (6.2843, 19.4938)
  line L604 (6.2843, 19.4938) -> (6.393, 19.3685)
  line L605 (6.393, 19.3685) -> (6.4859, 19.2337)
  line L606 (6.4859, 19.2337) -> (6.5355, 19.1682)
  line L607 (6.5355, 19.1682) -> (6.5898, 19.1054)
  line L608 (6.5898, 19.1054) -> (6.6498, 19.0459)
  line L609 (6.6498, 19.0459) -> (6.7176, 18.9909)
  line L610 (6.7176, 18.9909) -> (6.7556, 18.9657)
  line L611 (6.7556, 18.9657) -> (6.7976, 18.9428)
  line L612 (6.7976, 18.9428) -> (6.8454, 18.9231)
  line L613 (6.8454, 18.9231) -> (6.9041, 18.9094)
  line L614 (6.9041, 18.9094) -> (7.0246, 18.9294)
  line L615 (7.0246, 18.9294) -> (7.4607, 19.1516)
  line L616 (7.4607, 19.1516) -> (7.5477, 19.2373)
  line L617 (7.5477, 19.2373) -> (7.5712, 19.2929)
  line L618 (7.5712, 19.2929) -> (7.5834, 19.3432)
  line L619 (7.5834, 19.3432) -> (7.5894, 19.3906)
  line L620 (7.5894, 19.3906) -> (7.5914, 19.4362)
  line L621 (7.5914, 19.4362) -> (7.5868, 19.5233)
  line L622 (7.5868, 19.5233) -> (7.5739, 19.6068)
  line L623 (7.5739, 19.6068) -> (7.555, 19.6877)
  line L624 (7.555, 19.6877) -> (7.5312, 19.7663)
  line L625 (7.5312, 19.7663) -> (7.4767, 19.9207)
  line L626 (7.4767, 19.9207) -> (7.4392, 20.0824)
  line L627 (7.4392, 20.0824) -> (7.4146, 20.2493)
  line L628 (7.4146, 20.2493) -> (7.4002, 20.4204)
  line L629 (7.4002, 20.4204) -> (7.3948, 20.5948)
  line L630 (7.3948, 20.5948) -> (7.3976, 20.7721)
  line L631 (7.3976, 20.7721) -> (7.4081, 20.952)
  line L632 (7.4081, 20.952) -> (7.426, 21.1341)
  line L633 (7.426, 21.1341) -> (7.4511, 21.3183)
  line L634 (7.4511, 21.3183) -> (7.4833, 21.5042)
  line L635 (7.4833, 21.5042) -> (7.5223, 21.6917)
  line L636 (7.5223, 21.6917) -> (7.556, 21.8333)
  line L637 (7.556, 21.8333) -> (7.9577, 21.9638)
  line L638 (7.9577, 21.9638) -> (8.0681, 21.8691)
  line L639 (8.0681, 21.8691) -> (8.2099, 21.7403)
  line L640 (8.2099, 21.7403) -> (8.3452, 21.6088)
  line L641 (8.3452, 21.6088) -> (8.4738, 21.4746)
  line L642 (8.4738, 21.4746) -> (8.5954, 21.3378)
  line L643 (8.5954, 21.3378) -> (8.7096, 21.1984)
  line L644 (8.7096, 21.1984) -> (8.8161, 21.0566)
  line L645 (8.8161, 21.0566) -> (8.9141, 20.9123)
  line L646 (8.9141, 20.9123) -> (9.003, 20.7655)
  line L647 (9.003, 20.7655) -> (9.0813, 20.6159)
  line L648 (9.0813, 20.6159) -> (9.146, 20.4631)
  line L649 (9.146, 20.4631) -> (9.1927, 20.3062)
  line L650 (9.1927, 20.3062) -> (9.2196, 20.2285)
  line L651 (9.2196, 20.2285) -> (9.2518, 20.152)
  line L652 (9.2518, 20.152) -> (9.2905, 20.0769)
  line L653 (9.2905, 20.0769) -> (9.338, 20.0037)
  line L654 (9.338, 20.0037) -> (9.3664, 19.968)
  line L655 (9.3664, 19.968) -> (9.3992, 19.9332)
  line L656 (9.3992, 19.9332) -> (9.4386, 19.8997)
  line L657 (9.4386, 19.8997) -> (9.4902, 19.8685)
  line L658 (9.4902, 19.8685) -> (9.611, 19.8503)
  line L659 (9.611, 19.8503) -> (10.0944, 19.9269)
  line L660 (10.0944, 19.9269) -> (10.2037, 19.9815)
  line L661 (10.2037, 19.9815) -> (10.2431, 20.0271)
  line L662 (10.2431, 20.0271) -> (10.2703, 20.0711)
  line L663 (10.2703, 20.0711) -> (10.2907, 20.1144)
  line L664 (10.2907, 20.1144) -> (10.3066, 20.1571)
  line L665 (10.3066, 20.1571) -> (10.3292, 20.2414)
  line L666 (10.3292, 20.2414) -> (10.3428, 20.3248)
  line L667 (10.3428, 20.3248) -> (10.3498, 20.4075)
  line L668 (10.3498, 20.4075) -> (10.3514, 20.4897)
  line L669 (10.3514, 20.4897) -> (10.3473, 20.6534)
  line L670 (10.3473, 20.6534) -> (10.3616, 20.8187)
  line L671 (10.3616, 20.8187) -> (10.3898, 20.9851)
  line L672 (10.3898, 20.9851) -> (10.429, 21.1522)
  line L673 (10.429, 21.1522) -> (10.4777, 21.3198)
  line L674 (10.4777, 21.3198) -> (10.5351, 21.4876)
  line L675 (10.5351, 21.4876) -> (10.6007, 21.6554)
  line L676 (10.6007, 21.6554) -> (10.6741, 21.823)
  line L677 (10.6741, 21.823) -> (10.7549, 21.9904)
  line L678 (10.7549, 21.9904) -> (10.8429, 22.1573)
  line L679 (10.8429, 22.1573) -> (10.9379, 22.3236)
  line L680 (10.9379, 22.3236) -> (11.0137, 22.4478)
  line L681 (11.0137, 22.4478) -> (11.4361, 22.4478)
  line L682 (11.4361, 22.4478) -> (11.5119, 22.3236)
  line L683 (11.5119, 22.3236) -> (11.6069, 22.1573)
  line L684 (11.6069, 22.1573) -> (11.695, 21.9904)
  line L685 (11.695, 21.9904) -> (11.7758, 21.823)
  line L686 (11.7758, 21.823) -> (11.8491, 21.6554)
  line L687 (11.8491, 21.6554) -> (11.9147, 21.4876)
  line L688 (11.9147, 21.4876) -> (11.9721, 21.3198)
  line L689 (11.9721, 21.3198) -> (12.0208, 21.1522)
  line L690 (12.0208, 21.1522) -> (12.06, 20.9851)
  line L691 (12.06, 20.9851) -> (12.0882, 20.8187)
  line L692 (12.0882, 20.8187) -> (12.1025, 20.6534)
  line L693 (12.1025, 20.6534) -> (12.0984, 20.4897)
  line L694 (12.0984, 20.4897) -> (12.1, 20.4075)
  line L695 (12.1, 20.4075) -> (12.107, 20.3248)
  line L696 (12.107, 20.3248) -> (12.1206, 20.2414)
  line L697 (12.1206, 20.2414) -> (12.1432, 20.1571)
  line L698 (12.1432, 20.1571) -> (12.1591, 20.1144)
  line L699 (12.1591, 20.1144) -> (12.1796, 20.0711)
  line L700 (12.1796, 20.0711) -> (12.2067, 20.0271)
  line L701 (12.2067, 20.0271) -> (12.2461, 19.9815)
  line L702 (12.2461, 19.9815) -> (12.3554, 19.9269)
  line L703 (12.3554, 19.9269) -> (12.8388, 19.8503)
  line L704 (12.8388, 19.8503) -> (12.9596, 19.8685)
  line L705 (12.9596, 19.8685) -> (13.0112, 19.8997)
  line L706 (13.0112, 19.8997) -> (13.0506, 19.9332)
  line L707 (13.0506, 19.9332) -> (13.0834, 19.968)
  line L708 (13.0834, 19.968) -> (13.1118, 20.0037)
  line L709 (13.1118, 20.0037) -> (13.1593, 20.0769)
  line L710 (13.1593, 20.0769) -> (13.198, 20.152)
  line L711 (13.198, 20.152) -> (13.2302, 20.2285)
  line L712 (13.2302, 20.2285) -> (13.2572, 20.3062)
  line L713 (13.2572, 20.3062) -> (13.3038, 20.4631)
  line L714 (13.3038, 20.4631) -> (13.3685, 20.6159)
  line L715 (13.3685, 20.6159) -> (13.4468, 20.7655)
  line L716 (13.4468, 20.7655) -> (13.5357, 20.9123)
  line L717 (13.5357, 20.9123) -> (13.6338, 21.0566)
  line L718 (13.6338, 21.0566) -> (13.7402, 21.1984)
  line L719 (13.7402, 21.1984) -> (13.8544, 21.3378)
  line L720 (13.8544, 21.3378) -> (13.976, 21.4746)
  line L721 (13.976, 21.4746) -> (14.1046, 21.6088)
  line L722 (14.1046, 21.6088) -> (14.2399, 21.7403)
  line L723 (14.2399, 21.7403) -> (14.3817, 21.8691)
  line L724 (14.3817, 21.8691) -> (14.4922, 21.9638)
  line L725 (14.4922, 21.9638) -> (14.8938, 21.8333)
  line L726 (14.8938, 21.8333) -> (14.9275, 21.6917)
  line L727 (14.9275, 21.6917) -> (14.9665, 21.5042)
  line L728 (14.9665, 21.5042) -> (14.9987, 21.3183)
  line L729 (14.9987, 21.3183) -> (15.0238, 21.1341)
  line L730 (15.0238, 21.1341) -> (15.0418, 20.952)
  line L731 (15.0418, 20.952) -> (15.0523, 20.7721)
  line L732 (15.0523, 20.7721) -> (15.055, 20.5948)
  line L733 (15.055, 20.5948) -> (15.0496, 20.4204)
  line L734 (15.0496, 20.4204) -> (15.0352, 20.2493)
  line L735 (15.0352, 20.2493) -> (15.0106, 20.0824)
  line L736 (15.0106, 20.0824) -> (14.9731, 19.9207)
  line L737 (14.9731, 19.9207) -> (14.9186, 19.7663)
  line L738 (14.9186, 19.7663) -> (14.8948, 19.6877)
  line L739 (14.8948, 19.6877) -> (14.8759, 19.6068)
  line L740 (14.8759, 19.6068) -> (14.863, 19.5233)
  line L741 (14.863, 19.5233) -> (14.8584, 19.4362)
  line L742 (14.8584, 19.4362) -> (14.8604, 19.3906)
  line L743 (14.8604, 19.3906) -> (14.8665, 19.3432)
  line L744 (14.8665, 19.3432) -> (14.8787, 19.2929)
  line L745 (14.8787, 19.2929) -> (14.9021, 19.2373)
  line L746 (14.9021, 19.2373) -> (14.9891, 19.1516)
  line L747 (14.9891, 19.1516) -> (15.4252, 18.9294)
  line L748 (15.4252, 18.9294) -> (15.5457, 18.9094)
  line L749 (15.5457, 18.9094) -> (15.6044, 18.9231)
  line L750 (15.6044, 18.9231) -> (15.6523, 18.9428)
  line L751 (15.6523, 18.9428) -> (15.6942, 18.9657)
  line L752 (15.6942, 18.9657) -> (15.7322, 18.9909)
  line L753 (15.7322, 18.9909) -> (15.8, 19.0459)
  line L754 (15.8, 19.0459) -> (15.8601, 19.1054)
  line L755 (15.8601, 19.1054) -> (15.9143, 19.1682)
  line L756 (15.9143, 19.1682) -> (15.964, 19.2337)
  line L757 (15.964, 19.2337) -> (16.0568, 19.3685)
  line L758 (16.0568, 19.3685) -> (16.1656, 19.4938)
  line L759 (16.1656, 19.4938) -> (16.2862, 19.6119)
  line L760 (16.2862, 19.6119) -> (16.4161, 19.7241)
  line L761 (16.4161, 19.7241) -> (16.554, 19.831)
  line L762 (16.554, 19.831) -> (16.6991, 19.933)
  line L763 (16.6991, 19.933) -> (16.8508, 20.0302)
  line L764 (16.8508, 20.0302) -> (17.0087, 20.1228)
  line L765 (17.0087, 20.1228) -> (17.1725, 20.2107)
  line L766 (17.1725, 20.2107) -> (17.3418, 20.294)
  line L767 (17.3418, 20.294) -> (17.5164, 20.3726)
  line L768 (17.5164, 20.3726) -> (17.6507, 20.4286)
  line L769 (17.6507, 20.4286) -> (17.9924, 20.1803)
  line L770 (17.9924, 20.1803) -> (17.9807, 20.0353)
  line L771 (17.9807, 20.0353) -> (17.9599, 19.8449)
  line L772 (17.9599, 19.8449) -> (17.933, 19.6581)
  line L773 (17.933, 19.6581) -> (17.9, 19.4752)
  line L774 (17.9, 19.4752) -> (17.8608, 19.2964)
  line L775 (17.8608, 19.2964) -> (17.8152, 19.1221)
  line L776 (17.8152, 19.1221) -> (17.763, 18.9526)
  line L777 (17.763, 18.9526) -> (17.7039, 18.7885)
  line L778 (17.7039, 18.7885) -> (17.6374, 18.6302)
  line L779 (17.6374, 18.6302) -> (17.5624, 18.479)
  line L780 (17.5624, 18.479) -> (17.4768, 18.3369)
  line L781 (17.4768, 18.3369) -> (17.3773, 18.2069)
  line L782 (17.3773, 18.2069) -> (17.3303, 18.1394)
  line L783 (17.3303, 18.1394) -> (17.2873, 18.0684)
  line L784 (17.2873, 18.0684) -> (17.2493, 17.9929)
  line L785 (17.2493, 17.9929) -> (17.218, 17.9114)
  line L786 (17.218, 17.9114) -> (17.2058, 17.8675)
  line L787 (17.2058, 17.8675) -> (17.1969, 17.8205)
  line L788 (17.1969, 17.8205) -> (17.193, 17.7689)
  line L789 (17.193, 17.7689) -> (17.1981, 17.7089)
  line L790 (17.1981, 17.7089) -> (17.2544, 17.6005)
  line L791 (17.2544, 17.6005) -> (17.6005, 17.2544)
  line L792 (17.6005, 17.2544) -> (17.7089, 17.1981)
  line L793 (17.7089, 17.1981) -> (17.7689, 17.193)
  line L794 (17.7689, 17.193) -> (17.8205, 17.1969)
  line L795 (17.8205, 17.1969) -> (17.8675, 17.2058)
  line L796 (17.8675, 17.2058) -> (17.9114, 17.218)
  line L797 (17.9114, 17.218) -> (17.9929, 17.2493)
  line L798 (17.9929, 17.2493) -> (18.0684, 17.2873)
  line L799 (18.0684, 17.2873) -> (18.1394, 17.3303)
  line L800 (18.1394, 17.3303) -> (18.2069, 17.3773)
  line L801 (18.2069, 17.3773) -> (18.3369, 17.4768)
  line L802 (18.3369, 17.4768) -> (18.479, 17.5624)
  line L803 (18.479, 17.5624) -> (18.6302, 17.6374)
  line L804 (18.6302, 17.6374) -> (18.7885, 17.7039)
  line L805 (18.7885, 17.7039) -> (18.9526, 17.763)
  line L806 (18.9526, 17.763) -> (19.1221, 17.8152)
  line L807 (19.1221, 17.8152) -> (19.2964, 17.8608)
  line L808 (19.2964, 17.8608) -> (19.4752, 17.9)
  line L809 (19.4752, 17.9) -> (19.6581, 17.933)
  line L810 (19.6581, 17.933) -> (19.8449, 17.9599)
  line L811 (19.8449, 17.9599) -> (20.0353, 17.9807)
  line L812 (20.0353, 17.9807) -> (20.1803, 17.9924)
  line L813 (20.1803, 17.9924) -> (20.4286, 17.6507)
  line L814 (20.4286, 17.6507) -> (20.3726, 17.5164)
  line L815 (20.3726, 17.5164) -> (20.294, 17.3418)
  line L816 (20.294, 17.3418) -> (20.2107, 17.1725)
  line L817 (20.2107, 17.1725) -> (20.1228, 17.0087)
  line L818 (20.1228, 17.0087) -> (20.0302, 16.8508)
  line L819 (20.0302, 16.8508) -> (19.933, 16.6991)
  line L820 (19.933, 16.6991) -> (19.831, 16.554)
  line L821 (19.831, 16.554) -> (19.7241, 16.4161)
  line L822 (19.7241, 16.4161) -> (19.6119, 16.2862)
  line L823 (19.6119, 16.2862) -> (19.4938, 16.1656)
  line L824 (19.4938, 16.1656) -> (19.3685, 16.0568)
  line L825 (19.3685, 16.0568) -> (19.2337, 15.964)
  line L826 (19.2337, 15.964) -> (19.1682, 15.9143)
  line L827 (19.1682, 15.9143) -> (19.1054, 15.8601)
  line L828 (19.1054, 15.8601) -> (19.0459, 15.8)
  line L829 (19.0459, 15.8) -> (18.9909, 15.7322)
  line L830 (18.9909, 15.7322) -> (18.9657, 15.6942)
  line L831 (18.9657, 15.6942) -> (18.9428, 15.6523)
  line L832 (18.9428, 15.6523) -> (18.9231, 15.6044)
  line L833 (18.9231, 15.6044) -> (18.9094, 15.5457)
  line L834 (18.9094, 15.5457) -> (18.9294, 15.4252)
  line L835 (18.9294, 15.4252) -> (19.1516, 14.9891)
  line L836 (19.1516, 14.9891) -> (19.2373, 14.9021)
  line L837 (19.2373, 14.9021) -> (19.2929, 14.8787)
  line L838 (19.2929, 14.8787) -> (19.3432, 14.8665)
  line L839 (19.3432, 14.8665) -> (19.3906, 14.8604)
  line L840 (19.3906, 14.8604) -> (19.4362, 14.8584)
  line L841 (19.4362, 14.8584) -> (19.5233, 14.863)
  line L842 (19.5233, 14.863) -> (19.6068, 14.8759)
  line L843 (19.6068, 14.8759) -> (19.6877, 14.8948)
  line L844 (19.6877, 14.8948) -> (19.7663, 14.9186)
  line L845 (19.7663, 14.9186) -> (19.9207, 14.9731)
  line L846 (19.9207, 14.9731) -> (20.0824, 15.0106)
  line L847 (20.0824, 15.0106) -> (20.2493, 15.0352)
  line L848 (20.2493, 15.0352) -> (20.4204, 15.0496)
  line L849 (20.4204, 15.0496) -> (20.5948, 15.055)
  line L850 (20.5948, 15.055) -> (20.7721, 15.0523)
  line L851 (20.7721, 15.0523) -> (20.952, 15.0418)
  line L852 (20.952, 15.0418) -> (21.1341, 15.0238)
  line L853 (21.1341, 15.0238) -> (21.3183, 14.9987)
  line L854 (21.3183, 14.9987) -> (21.5042, 14.9665)
  line L855 (21.5042, 14.9665) -> (21.6917, 14.9275)
  line L856 (21.6917, 14.9275) -> (21.8333, 14.8938)
  line L857 (21.8333, 14.8938) -> (21.9638, 14.4922)
  line L858 (21.9638, 14.4922) -> (21.8691, 14.3817)
  line L859 (21.8691, 14.3817) -> (21.7403, 14.2399)
  line L860 (21.7403, 14.2399) -> (21.6088, 14.1046)
  line L861 (21.6088, 14.1046) -> (21.4746, 13.976)
  line L862 (21.4746, 13.976) -> (21.3378, 13.8544)
  line L863 (21.3378, 13.8544) -> (21.1984, 13.7402)
  line L864 (21.1984, 13.7402) -> (21.0566, 13.6338)
  line L865 (21.0566, 13.6338) -> (20.9123, 13.5357)
  line L866 (20.9123, 13.5357) -> (20.7655, 13.4468)
  line L867 (20.7655, 13.4468) -> (20.6159, 13.3685)
  line L868 (20.6159, 13.3685) -> (20.4631, 13.3038)
  line L869 (20.4631, 13.3038) -> (20.3062, 13.2572)
  line L870 (20.3062, 13.2572) -> (20.2285, 13.2302)
  line L871 (20.2285, 13.2302) -> (20.152, 13.198)
  line L872 (20.152, 13.198) -> (20.0769, 13.1593)
  line L873 (20.0769, 13.1593) -> (20.0037, 13.1118)
  line L874 (20.0037, 13.1118) -> (19.968, 13.0834)
  line L875 (19.968, 13.0834) -> (19.9332, 13.0506)
  line L876 (19.9332, 13.0506) -> (19.8997, 13.0112)
  line L877 (19.8997, 13.0112) -> (19.8685, 12.9596)
  line L878 (19.8685, 12.9596) -> (19.8503, 12.8388)
  line L879 (19.8503, 12.8388) -> (19.9269, 12.3554)
  circle A0 centre (11.2249, 11.2249) radius 0.5
  point P0 (0, 0)
  constraints: 1760 end point, 1 centre point
extrude "Extrusion1" add sketch "Sketch1" along normal blind 5
sketch "Sketch2" plane through (0, 0, 0) normal (0, -1, 0) x (1, 0, 0)
  arc A0 (-8.9644, 10.5805) -> (-8.8759, 11.1392) centre (-9.1995, 10.9041) ccw projected
  line L0 (-8.8759, 11.1392) -> (-10.5805, 13.4854) projected
  arc A1 (-10.5805, 13.4854) -> (-11.1392, 13.5739) centre (-10.9041, 13.2503) ccw projected
  line L1 (-11.1392, 13.5739) -> (-13.4854, 11.8693) projected
  arc A2 (-13.4854, 11.8693) -> (-13.5739, 11.3106) centre (-13.2503, 11.5457) ccw projected
  line L2 (-13.5739, 11.3106) -> (-11.8693, 8.9644) projected
  arc A3 (-11.8693, 8.9644) -> (-11.3106, 8.8759) centre (-11.5457, 9.1995) ccw projected
  line L3 (-11.3106, 8.8759) -> (-8.9644, 10.5805) projected
  circle A4 centre (-11.2249, 11.2249) radius 6.5 projected
  point P0 (0, 0)
extrude "Extrusion2" cut sketch "Sketch2" against normal up to next contours L3 A3 L2 A2 L1 A1 L0 A0
body "Solid2"
